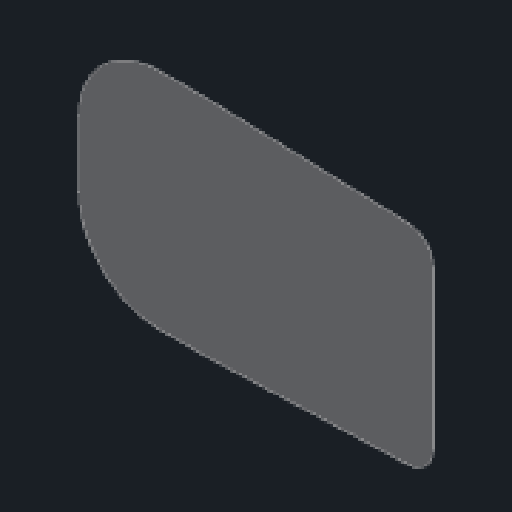
# Autodesk Inventor part: CHAPA_6
Saved by Autodesk Inventor 2024.3 (Build 283343000, 343)
## iProperties
Created: 2024-06-30
Part Number: CHAPA_6
Material: Generic
Document SubType Name: Sheet Metal
Designer: Niler
Density: 1 g/cm^3
Sheet Metal Rule: Default_mm
Appearance: Default
Author: Niler
Autodesk Inventor part; units mm, degrees
ref_plane "YZ Plane" through (0, 0, 0) normal (1, 0, 0) x (0, 1, 0)
ref_plane "XZ Plane" through (0, 0, 0) normal (0, 1, 0) x (-1, 0, 0)
ref_plane "XY Plane" through (0, 0, 0) normal (0, 0, 1) x (1, 0, 0)
sketch "Sketch1" plane through (0, 0, 0) normal (0, 0, 1) x (1, 0, 0)
  arc A0 (216.4448, 899.4448) -> (-166.5552, 516.4448) centre (216.4448, 516.4448) ccw
  line L0 (-166.5552, 216.4448) -> (-166.5552, 516.4448)
  arc A1 (-166.5552, 216.4448) -> (216.4448, -166.5552) centre (216.4448, 216.4448) ccw
  line L1 (443.4448, -166.5552) -> (216.4448, -166.5552)
  line L2 (216.4448, 899.4448) -> (443.4448, 899.4448)
  line L3 (443.5712, 899.4425) -> (1403.908, 864.732)
  line L4 (1403.908, -131.8425) -> (443.5712, -166.5529)
  arc A2 (443.4448, -166.5552) -> (443.5712, -166.5529) centre (443.4448, -163.0552) ccw
  arc A3 (443.5712, 899.4425) -> (443.4448, 899.4448) centre (443.4448, 895.9448) ccw
  arc A4 (1521.5977, 742.7757) -> (1403.908, 864.732) centre (1399.4977, 742.7117) ccw
  line L5 (1521.5977, 742.7757) -> (1521.6067, 725.4805)
  line L6 (1521.6067, 7.4091) -> (1521.5977, -9.8861)
  arc A5 (1403.908, -131.8425) -> (1521.5977, -9.8861) centre (1399.4977, -9.8222) ccw
  line L7 (1521.6067, 725.4805) -> (1521.6067, 7.4091)
  point P0 (0, 0)
extrude "Plate1" add sketch "Sketch1" along normal blind 1.5
equation "\"d0\" = Thickness"
equation "\"BendRadius\" = Thickness"
equation "\"BendReliefWidth\" = Thickness"
equation "\"BendReliefDepth\" = 0.5 * Thickness"
equation "\"CornerReliefSize\" = 4 * Thickness"
equation "\"MinimumRemnant\" = 2 * Thickness"
equation "\"TransitionRadius\" = BendRadius"
equation "\"JacobiRadiusSize\" = BendRadius"
equation "\"GapSize\" = Thickness"
equation "\"Thickness\" = 1.5"
body "Solid1"
